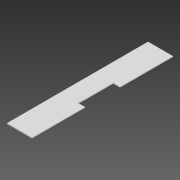
# Autodesk Inventor part: border2
Saved by Autodesk Inventor 2020 (Build 240168000, 168)
## iProperties
Created: 2022-08-25
Part Number: border2
Material: Generic
Document SubType Name: Modeling
Designer: Umair
Density: 1 g/cm^3
Appearance: Default
Author: Umair
Autodesk Inventor part; units mm, degrees
ref_plane "YZ Plane" through (0, 0, 0) normal (1, 0, 0) x (0, 1, 0)
ref_plane "XZ Plane" through (0, 0, 0) normal (0, 1, 0) x (-1, 0, 0)
ref_plane "XY Plane" through (0, 0, 0) normal (0, 0, 1) x (1, 0, 0)
sketch "Sketch1" plane through (0, 0, 0) normal (0, 1, 0) x (-1, 0, 0)
  line L0 (55, 312.5) -> (-55, 312.5)
  line L1 (-55, 312.5) -> (-55, -312.5)
  line L2 (-55, -312.5) -> (55, -312.5)
  line L3 (55, -312.5) -> (55, 312.5)
  line L4 (55, 312.5) -> (-55, -312.5) construction
  line L5 (-55, 312.5) -> (55, -312.5) construction
  line L6 (0, 0) -> (-55, 0)
  line L7 (-55, 0) -> (-25, 0)
  line L8 (-25, 0) -> (-25, -78)
  line L9 (-25, -78) -> (-25, 78)
  line L10 (-25, 78) -> (-55, 78)
  line L11 (-25, -78) -> (-55, -78)
  dimension "d0" = 110
  dimension "d1" = 625
  dimension "d2" = 30
  dimension "d3" = 78
  dimension "d4" = 156
  constraints: 24 end point, 4 perpendicular, 4 point on line, 3 midpoint, 2 parallel, 1 horizontal
  measures "d0" distance of L2.end L1.end
  measures "d1" distance of L1.end L0.end
  measures "d2" distance of L6.end L7.end
  measures "d3" distance of L7.end L8.end
  measures "d4" distance of L8.end L9.end
extrude "Extrusion1" add sketch "Sketch1" along normal blind 3 contours L3 L2 L1 L11 L8 L9 L10 L0
body "Solid1"
